Autodesk Inventor part; units mm, degrees
(part 2 of 2)
  arc A631 (-4.6561, 92.6487) -> (-5.7499, 92.5872) centre (0, 0) ccw
  arc A632 (-3.4438, 89.6341) -> (-4.6561, 92.6487) centre (-22.5209, 83.7138) ccw
  arc A633 (-2.385, 89.6685) -> (-3.4438, 89.6341) centre (0, 0) ccw
  arc A634 (-1.3711, 92.7554) -> (-2.385, 89.6685) centre (17.0363, 84.9998) ccw
  arc A635 (-0.2756, 92.7652) -> (-1.3711, 92.7554) centre (0, 0) ccw
  arc A636 (0.7929, 89.6967) -> (-0.2756, 92.7652) centre (-18.5425, 84.684) ccw
  arc A637 (1.8522, 89.6811) -> (0.7929, 89.6967) centre (0, 0) ccw
  arc A638 (3.0107, 92.7167) -> (1.8522, 89.6811) centre (21.0314, 84.1004) ccw
  arc A639 (4.1055, 92.6747) -> (3.0107, 92.7167) centre (0, 0) ccw
  circle A640 centre (0, 0) radius 102.0421
  point P0 (-3.4869, 89.7711)
  point P1 (-3.4231, 89.6349)
  point P2 (1.8314, 89.6815)
  point P3 (1.8928, 89.8188)
  constraints: 1280 point on circle, 641 centre point
extrude "Extrusion1" add sketch "Sketch2" along normal blind 5 contours A107 A106 A105 A104 A103 A102 A101 A100 A99 A98 A97 A96 A95 A94 A93 A92 A91 A90 A89 A88 A87 A86 A85 A84 A83 A82 A81 A80 A79 A78 A77 A76 A75 A74 A73 A72 A71 A70 A69 A68 A67 A66 A65 A64 A63 A62 A61 A60 A59 A58 A57 A56 A55 A54 A53 A52 A51 A50 A49 A48 A47 A46 A45 A44 A43 A42 A41 A40 A39 A38 A37 A36 A35 A34 A33 A32 A31 A30 A29 A28 A27 A26 A25 A24 A23 A22 A21 A20 A19 A18 A17 A16 A15 A14 A13 A12 A11 A10 A9 A8 A632 A633 A7 A6 A5 A4 A3 A2 A637 A638 A1 A0 | A640
body "Solid1"
